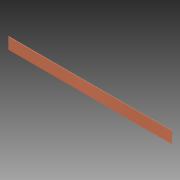
# Autodesk Inventor part: rfPlateShort
Saved by Autodesk Inventor 2015 SP1 (Build 190203100, 203)
## iProperties
Created: 2011-06-08
Part Number: rfPlateShort
Document SubType Name: Modeling
Designer: ijs09
Density: 1 g/cm^3
Material: Generic
Appearance: Default
Author: ijs09
Autodesk Inventor part; units mm, degrees
ref_plane "YZ Plane" through (0, 0, 0) normal (1, 0, 0) x (0, 1, 0)
ref_plane "XZ Plane" through (0, 0, 0) normal (0, 1, 0) x (-1, 0, 0)
ref_plane "XY Plane" through (0, 0, 0) normal (0, 0, 1) x (1, 0, 0)
sketch "Sketch2" plane through (0, 0, 0) normal (0, 1, 0) x (-1, 0, 0)
  line L0 (-400, 28) -> (400, 28)
  line L1 (400, 28) -> (400, -28)
  line L2 (400, -28) -> (-400, -28)
  line L3 (-400, -28) -> (-400, 28)
  point P0 (0, 0)
  dimension "d0" = 56
  dimension "d1" = 28
  dimension "d2" = 800
  dimension "d3" = 400
  constraints: 8 end point, 2 parallel, 1 horizontal, 1 perpendicular
  measures "d0" distance between parallel lines of L0 L2
  measures "d1" distance from line of point (0, 0) L0
  measures "d2" distance between parallel lines of L3 L1
  measures "d3" distance from line of point (0, 0) L3
extrude "Extrusion1" add sketch "Sketch2" along normal blind 2
sketch "Sketch3" plane through (0, 0, 0) normal (0, -1, 0) x (1, 0, 0)
  circle A0 centre (-396.5, 0) radius 1.15
  line L0 (-400, 28) -> (-400, -28) projected
  point P0 (0, 0)
  dimension "d6" = 2.3
  dimension "d7" = 3.5
  constraints: 1 centre point
  measures "d6" diameter of A0
  measures "d7" distance from line of A0.centre L0
hole "Hole1" at (-396.5, 0, 0) direction (0, 1, 0) diameter 2.3 end through all
sketch "Sketch4" plane through (0, 0, 0) normal (0, -1, 0) x (1, 0, 0)
  circle A0 centre (396.5, 0) radius 1.15
  line L0 (400, -28) -> (400, 28) projected
  point P0 (0, 0)
  dimension "d15" = 2.3
  dimension "d16" = 3.5
  constraints: 1 centre point
  measures "d15" diameter of A0
  measures "d16" distance from line of L0 A0.centre
hole "Hole2" at (396.5, 0, 0) direction (0, 1, 0) diameter 2.3 end through all
equation "\"d1\" = 0.5 * d0"
equation "\"d3\" = 0.5 * d2"
body "Solid1"
